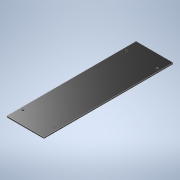
# Autodesk Inventor part: 三段目アクリル板
Saved by Autodesk Inventor 2022 (Build 260153000, 153)
## iProperties
Created: 2022-12-07
Part Number: 三段目アクリル板
Material: ABS プラスチック
Document SubType Name: Modeling
Designer: tdn82
Density: 1.06 g/cm^3
Appearance: 光沢 - 黒
Author: tdn82
Autodesk Inventor part; units mm, degrees
ref_plane "YZ Plane" through (0, 0, 0) normal (1, 0, 0) x (0, 1, 0)
ref_plane "XZ Plane" through (0, 0, 0) normal (0, 1, 0) x (-1, 0, 0)
ref_plane "XY Plane" through (0, 0, 0) normal (0, 0, 1) x (1, 0, 0)
sketch "スケッチ1" plane through (0, 0, 0) normal (0, 1, 0) x (-1, 0, 0)
  line L0 (0, 0) -> (-57.5, 0)
  line L1 (-57.5, 0) -> (-57.5, -200)
  line L2 (-57.5, -200) -> (0, -200)
  line L3 (0, -200) -> (0, 0)
  dimension "d0" = 200
  dimension "d1" = 57.5
  constraints: 8 end point, 2 parallel, 1 horizontal, 1 perpendicular
  measures "d0" distance of L2.end L0.start
  measures "d1" distance of L0.start L0.end
extrude "押し出し1" add sketch "スケッチ1" along normal blind 2
sketch "スケッチ3" plane through (0, 0, 0) normal (0, -1, 0) x (1, 0, 0)
  line L0 (57.5, 0) -> (57.5, -200) projected
  line L1 (57.5, -200) -> (0, -200) projected
  line L2 (0, -200) -> (0, 0) projected
  point P0 (52.5, -20)
  point P1 (52.5, -180)
  point P2 (5, -180)
  point P3 (5, -20)
  dimension "d4" = 5
  dimension "d5" = 180
  dimension "d6" = 160
  dimension "d17" = 5
  dimension "d18" = 5
  dimension "d19" = 5
  dimension "d20" = 47.5
  measures "d4" distance from line of point (52.5, -20) L0
  measures "d5" distance from line of point (52.5, -20) L1
  measures "d6" distance of point (52.5, -180) point (52.5, -20)
  measures "d17" distance from line of L2 point (5, -180)
  measures "d18" distance from line of point (5, -20) L2
  measures "d19" distance from line of L0 point (52.5, -180)
  measures "d20" distance of point (52.5, -180) point (5, -180)
hole "穴1" at (52.5, 0, -20) at (52.5, 0, -180) at (5, 0, -180) at (5, 0, -20) direction (0, 1, 0) diameter 3 end through all
